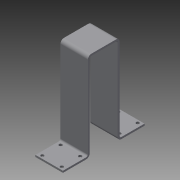
# Autodesk Inventor part: Sheet Metal Arm
Saved by Autodesk Inventor 2015 (Build 190159000, 159)
## iProperties
Created: 2015-02-24
Part Number: Sheet Metal Arm
Material: Generic
Document SubType Name: Sheet Metal
Designer: pltwe4
Density: 1 g/cm^3
Sheet Metal Rule: Default_mm
Appearance: Default
Author: pltwe4
Autodesk Inventor part; units mm, degrees
ref_plane "YZ Plane" through (0, 0, 0) normal (1, 0, 0) x (0, 1, 0)
ref_plane "XZ Plane" through (0, 0, 0) normal (0, 1, 0) x (-1, 0, 0)
ref_plane "XY Plane" through (0, 0, 0) normal (0, 0, 1) x (1, 0, 0)
sketch "Sketch1" plane through (0, 0, 0) normal (0, 1, 0) x (-1, 0, 0)
  line L0 (24, 219) -> (-24, 219)
  line L1 (-24, 219) -> (-24, -219)
  line L2 (-24, -219) -> (24, -219)
  line L3 (24, -219) -> (24, 219)
  line L4 (0, -306.6) -> (0, 306.6) projected
  line L5 (-33.6, 0) -> (33.6, 0) projected
  circle A0 centre (17, 214) radius 2.75
  circle A1 centre (17, 182) radius 2.75
  circle A2 centre (-17, 214) radius 2.75
  circle A3 centre (-17, 182) radius 2.75
  circle A4 centre (17, -182) radius 2.75
  circle A5 centre (17, -214) radius 2.75
  circle A6 centre (-17, -182) radius 2.75
  circle A7 centre (-17, -214) radius 2.75
  line L6 (24, 175) -> (-24, 175)
  line L7 (24, 25) -> (-24, 25)
  line L8 (24, -25) -> (-24, -25)
  line L9 (24, -175) -> (-24, -175)
  point P0 (0, 0)
  dimension "d1" = 48
  dimension "d2" = 34
  dimension "d3" = 32
  dimension "d4" = 5
  dimension "d5" = 5.5
  dimension "d6" = 34
  dimension "d7" = 50
  dimension "d8" = 44
  dimension "d9" = 44
  dimension "d10" = 150
  constraints: 16 end point, 8 centre point, 8 point on line, 4 perpendicular, 3 parallel, 1 equal radius, 1 horizontal, 9 other
  measures "d1" distance of L1.end L2.end
  measures "d2" distance of A2.centre A0.centre
  measures "d3" distance of A1.centre A0.centre
  measures "d4" distance from line of L0 A0.centre
  measures "d5" diameter of A0
  measures "d6" distance of A3.centre A1.centre
  measures "d7" distance between parallel lines of L8 L7
  measures "d8" distance between parallel lines of L0 L6
  measures "d9" distance between parallel lines of L9 L2
  measures "d10" distance between parallel lines of L8 L9
extrude "Plate1" add sketch "Sketch1" along normal blind 3.175
fold "Fold1" angle 90 bend radius 3.175 thickness 3.175 k factor 0.44 line from (-24, 0, 175) to (24, 0, 175) line at bend centre moving side (0, 0, 1) folds toward (0, 1, 0)
fold "Fold2" angle 90 bend radius 3.175 thickness 3.175 k factor 0.44 line from (-24, 0, 25) to (24, 0, 25) line at bend centre moving side (0, 0, 1) folds toward (0, -1, 0)
fold "Fold3" angle 90 bend radius 3.175 thickness 3.175 k factor 0.44 line from (-24, 0, -25) to (24, 0, -25) line at bend centre moving side (0, 0, 1) folds toward (0, -1, 0)
fold "Fold4" angle 90 bend radius 3.175 thickness 3.175 k factor 0.44 line from (-24, 0, -175) to (24, 0, -175) line at bend centre moving side (0, 0, 1) folds toward (0, 1, 0)
equation "\"d9\" = d8"
equation "\"d12\" = BendReliefWidth"
equation "\"d13\" = BendReliefDepth"
equation "\"d14\" = MinimumRemnant"
equation "\"d15\" = BendRadius"
equation "\"d17\" = BendRadius"
equation "\"d18\" = BendReliefWidth"
equation "\"d19\" = BendReliefDepth"
equation "\"d20\" = MinimumRemnant"
equation "\"d21\" = BendRadius"
equation "\"d23\" = BendRadius"
equation "\"d24\" = BendReliefWidth"
equation "\"d25\" = BendReliefDepth"
equation "\"d26\" = MinimumRemnant"
equation "\"d27\" = BendRadius"
equation "\"d29\" = BendRadius"
equation "\"d30\" = BendReliefWidth"
equation "\"d31\" = BendReliefDepth"
equation "\"d32\" = MinimumRemnant"
equation "\"d33\" = BendRadius"
equation "\"d35\" = BendRadius"
equation "\"BendRadius\" = Thickness"
equation "\"BendReliefWidth\" = Thickness"
equation "\"BendReliefDepth\" = 0.5 * Thickness"
equation "\"CornerReliefSize\" = 4 * Thickness"
equation "\"MinimumRemnant\" = 2 * Thickness"
equation "\"TransitionRadius\" = BendRadius"
equation "\"JacobiRadiusSize\" = BendRadius"
equation "\"GapSize\" = Thickness"
equation "\"d11\" = BendRadius"
equation "\"Thickness\" = 3.175"
body "Solid1"
